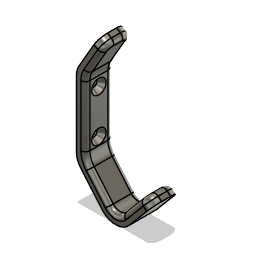
Coat Hook v2 (Autodesk Fusion 360 design; units mm, degrees)
Autodesk Fusion 360 part; units mm, degrees
sketch "Sketch1" plane through (0, 0, 0) normal (0, 0, 1) x (1, 0, 0)
  line L0 (0, 0) -> (0, 40)
  line L1 (0, 40) -> (11.547, 60)
  line L2 (0, 0) -> (12.9518, -15.4353)
  line L3 (20.6122, -15.4353) -> (33.4244, -0.1663)
  line L4 (33.4244, -0.1663) -> (37.2546, -3.3803)
  line L5 (7.2169, 62.5) -> (11.547, 60)
  arc A0 (12.9518, -15.4353) -> (20.6122, -15.4353) centre (16.782, -12.2214) ccw
  line L6 (24.4424, -18.6493) -> (37.2546, -3.3803)
  arc A1 (9.1215, -18.6493) -> (24.4424, -18.6493) centre (16.782, -12.2214) ccw
  line L7 (-5, -1.8199) -> (9.1215, -18.6493)
  line L8 (-5, -1.8199) -> (-5, 41.3397)
  line L9 (-5, 41.3397) -> (7.2169, 62.5)
  point P0 (16.782, -20)
  dimension "d1" = 20
  dimension "d2" = 40
  dimension "d4" = 140
  dimension "d5" = 20
  dimension "d8" = 80
  dimension "d9" = -5
  dimension "d10" = 5
  constraint coincident L0.start L2.start
  constraint vertical L0
  constraint perpendicular L1 L5
  constraint coincident P0 L2
  constraint coincident P0 L3
  constraint tangent L2 A0
  constraint tangent L3 A0
  measures "d1" vertical distance of L0.end L1.end
  measures "d2" distance of L0.start L0.end
  measures "d4" angle of L0 L2
  measures "d5" vertical distance of L0.start P0
  measures "d8" angle of L2 L3
  measures "d10" radius of A0
extrude "Extrude1" add sketch "Sketch1" along normal blind 10
sketch "Sketch2" plane through (0, 0, 0) normal (0, 0, 1) x (1, 0, 0)
sketch "Sketch3" plane through (0, 0, 0) normal (1, 0, 0) x (0, 0, -1)
extrude "Extrude2" add 1 faces at (-3.3333, 13.1733, 10) along direction (0, 0, 1) blind 5
sketch "Sketch4" plane through (0, 0, 0) normal (1, 0, 0) x (0, 0, -1)
  line L0 (0, 0) -> (0, 40)
  line L1 (0, 40) -> (-15, 40)
  line L2 (-15, 40) -> (-15, 0)
  line L3 (-15, 0) -> (0, 0)
  line L4 (-7.5, 40) -> (-7.5, 0) construction
  line L5 (-15, 20) -> (0, 20) construction
  circle A0 centre (-7.5, 32) radius 4
  circle A1 centre (-7.5, 8) radius 4
  dimension "d17" = 8
  dimension "d18" = 8
  constraint midpoint L1 L4.start
  constraint midpoint L3 L4.end
  constraint midpoint L2 L5.start
  constraint midpoint L0 L5.end
  constraint coincident L4 A0.centre
  constraint symmetric L5 A0 A1
  measures "d17" diameter of A0
  measures "d18" distance of L4.start A0.centre
extrude "Extrude3" cut sketch "Sketch4" against normal blind 15 contours A0 | A1
sketch "Sketch5" plane through (0, 0, 0) normal (1, 0, 0) x (0, 0, -1)
fillet "Fillet1" radius 5 1 edges at (35.3395, -1.7733, 15)
sketch "Sketch6" plane through (0, 0, 0) normal (1, 0, 0) x (0, 0, -1)
sketch "Sketch7" plane through (13.7283, 16.3607, 0) normal (0.642788, 0.766044, 0) x (0, 0, -1)
fillet "Fillet2" radius 5 1 edges at (35.3395, -1.7733, 0)
move_body "Move1" bodies 1 to x (1, 0, 0) y (0, 1, 0) z (0, 0, 1) at (-0.0992, 0, 0.3516)
delete_face "DeleteFace1" 1 faces at (-1.7658, 7.6017, 3.8715)
delete_face "DeleteFace2" 1 faces at (-3.4325, 31.6017, 3.8715)
sketch "Sketch8" plane through (0, 0, 0) normal (1, 0, 0) x (0, 0, -1)
sketch "Sketch9" plane through (-0.0992, 0, 0) normal (1, 0, 0) x (0, 0, -1)
  line L0 (-0.3516, 0) -> (-0.3516, 40)
  line L1 (-0.3516, 40) -> (-15.3516, 40)
  line L2 (-15.3516, 40) -> (-15.3516, 0)
  line L3 (-15.3516, 0) -> (-0.3516, 0)
  circle A0 centre (-7.8516, 32) radius 4
  circle A1 centre (-7.8516, 8) radius 4
  dimension "d25" = 8
  measures "d25" diameter of A0
extrude "Extrude4" cut sketch "Sketch9" against normal blind 3 draft -35 contours A0 | A1
extrude "Extrude5" cut 2 faces at (-3.0992, 8.2747, 8.422) (-3.0992, 32.244, 7.7107) along direction (-1, 0, 0) blind 5
fillet "Fillet3" radius 5 2 edges at (9.2828, 61.25, 15.3516) (9.2828, 61.25, 0.3516)
fillet "Fillet4" radius 10 4 edges at (-0.0992, 40, 7.8516) (-5.0992, 41.3397, 7.8516) (-5.0992, -1.8199, 7.8516) (-0.0992, 0, 7.8516)
fillet "Fillet5" radius 2.5 20 edges at (0.2416, 39.9087, 15.3516) (5.0942, 48.9952, 15.3516) (10.7156, 58.7317, 13.8871) (11.4479, 60, 7.8516) (10.7156, 58.7317, 1.816) (5.0942, 48.9952, 0.3516) (0.2416, 39.9087, 0.3516) (-0.0992, 20.4801, 0.3516) (0.5039, 0.2195, 0.3516) (7.5465, -9.1117, 0.3516) (16.6828, -17.2214, 0.3516) (25.3122, -9.7159, 0.3516) (32.3839, -1.2882, 1.816) (33.3253, -0.1663, 7.8516) (32.3839, -1.2882, 13.8871) (25.3122, -9.7159, 15.3516) (16.6828, -17.2214, 15.3516) (7.5465, -9.1117, 15.3516) (0.5039, 0.2195, 15.3516) (-0.0992, 20.4801, 15.3516)
